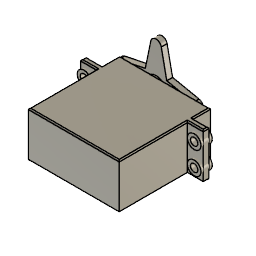
ASM of One of the legs (Autodesk Fusion 360 archive; units mm, degrees)
design "Servo MG996R Hosyond v2"
Autodesk Fusion 360 part; units mm, degrees
sketch "Sketch1" plane through (0, 0, 0) normal (0, 1, 0) x (1, 0, 0) in component "Servo Body"
  line L0 (20, 10) -> (-20, 10)
  line L1 (-20, 10) -> (-20, -10)
  line L2 (-20, -10) -> (20, -10)
  line L3 (20, -10) -> (20, 10)
  line L4 (20, 10) -> (-20, -10) construction
  line L5 (-20, 10) -> (20, -10) construction
  dimension "d20" = 40
  dimension "d21" = 20
  constraint horizontal L0
  constraint perpendicular L0 L1
  constraint parallel L0 L2
  constraint parallel L1 L3
  constraint coincident L4 origin
  constraint coincident L5 origin
  measures "d20" distance of L1.end L2.end
  measures "d21" distance of L0.end L1.end
extrude "Extrude1" add sketch "Sketch1" along normal blind 40.2 makes body 1 in component "Servo Body"
sketch "Sketch2" plane through (0, 40.2, 0) normal (0, 1, 0) x (-1, 0, 0) in component "Servo Body"
  line L0 (-20, 10) -> (-20, -10) construction
  line L1 (20, -10) -> (20, 10) construction
  line L2 (-20, 0) -> (20, 0) construction
  circle A0 centre (10, 0) radius 6.5
  circle A1 centre (10, 0) radius 2.9
  dimension "d24" = 10
  dimension "d25" = 13
  dimension "d26" = 5.8
  constraint midpoint L0 L2.start
  constraint midpoint L1 L2.end
  constraint coincident L2 A0.centre
  constraint concentric A0 A1
  measures "d24" distance of L2.end A0.centre
  measures "d25" diameter of A0
  measures "d26" diameter of A1
extrude "Extrude2" add sketch "Sketch2" along normal blind 2 contours A0 | A1 bodies 1 in component "Servo Body"
extrude "Extrude3" add sketch "Sketch2" along normal blind 6 contours A1 bodies 1 in component "Servo Body"
sketch "Sketch3" plane through (20, 0, 0) normal (1, 0, 0) x (0, 1, 0) in component "Servo Body"
  line L0 (30, 10) -> (32.5, 10)
  line L1 (32.5, 10) -> (32.5, -10)
  line L2 (32.5, -10) -> (30, -10)
  line L3 (30, -10) -> (30, 10)
  line L4 (0, 10) -> (40.2, 10)
  line L5 (0, -10) -> (40.2, -10)
  dimension "d31" = 2.5
  dimension "d32" = 30
  constraint horizontal L0
  constraint vertical L1
  constraint horizontal L2
  constraint vertical L3
  constraint coincident L1.end L5
  constraint coincident L0.start L4
  measures "d31" distance of L0.start L0.end
  measures "d32" distance of L0.start L4.start
extrude "Extrude4" add sketch "Sketch3" along normal blind 7 bodies 1 in component "Servo Body"
extrude "Extrude5" add sketch "Sketch3" against normal blind 7 from surface at -40 bodies 1 in component "Servo Body"
sketch "Sketch4" plane through (0, 32.5, 0) normal (0, 1, 0) x (-1, 0, 0) in component "Servo Body"
  circle A0 centre (24.25, -5) radius 2.22
  circle A1 centre (-24.25, -5) radius 2.22
  line L0 (20, -10) -> (27, -10)
  line L1 (20, 10) -> (27, 10)
  line L2 (-20, -10) -> (-27, -10)
  line L3 (-20, 10) -> (-27, 10)
  circle A2 centre (24.25, 5) radius 2.22
  circle A3 centre (-24.25, 5) radius 2.22
  line L4 (24.25, -5) -> (-24.25, -5) construction
  line L5 (-24.25, -5) -> (-24.25, 5) construction
  line L6 (-24.25, 5) -> (24.25, 5) construction
  line L7 (24.25, 5) -> (24.25, -5) construction
  line L8 (24.25, -5) -> (-24.25, 5) construction
  line L9 (-24.25, -5) -> (24.25, 5) construction
  line L10 (24.25, 0) -> (24.25, -10) construction
  dimension "d38" = 4.44
  dimension "d44" = 48.5
  constraint equal A0 A1
  constraint horizontal A0.centre A1.centre
  constraint equal A0 A2
  constraint equal A1 A3
  constraint horizontal L4
  constraint perpendicular L4 L5
  constraint parallel L4 L6
  constraint parallel L5 L7
  constraint coincident L8 origin
  constraint coincident L9 origin
  constraint coincident A0.centre L4.start
  constraint coincident A3.centre L5.end
  constraint coincident A2.centre L6.end
  constraint coincident A1.centre L4.end
  constraint midpoint L7 L10.start
  constraint coincident L0 L10.end
  constraint perpendicular L0 L10
  constraint midpoint A0.centre L10
  measures "d38" diameter of A0
  measures "d44" distance of A0.centre A1.centre
extrude "Extrude6" cut sketch "Sketch4" against normal up to surface (2.5 mm away) bodies 1 in component "Servo Body"
ref_plane "WorkPlane1" through (-10, 42.45, 0) normal (0, 1, 0) x (-1, 0, 0) in component "Connector"
sketch "Sketch1 (2)" plane through (0, 42.45, 0) normal (0, 1, 0) x (1, 0, 0) in component "Connector"
  arc A0 (-10, -18.3) -> (-7.6779, -16.4093) centre (-10, -15.9287) ccw
  line L0 (-5.2624, -4.7376) -> (-7.6779, -16.4093)
  line L1 (5.9287, 0) -> (6.4093, -2.3221) construction
  line L2 (-7.6779, -16.4093) -> (-10, -15.9287) construction
  arc A1 (6.4093, -2.3221) -> (8.3, 0) centre (5.9287, 0) ccw
  line L3 (-10, 0) -> (5.9287, 0) construction
  line L4 (6.4093, -2.3221) -> (-5.2624, -4.7376)
  line L5 (-5.2624, -4.7376) -> (-10, 0) construction
  line L6 (-10, -15.9287) -> (-10, -18.3) construction
  line L7 (5.9287, 0) -> (8.3, 0) construction
  line L8 (-10, -15.9287) -> (-10, 0) construction
  circle A2 centre (-10, 0) radius 4.35
  circle A3 centre (-10, 0) radius 2.9
  arc A4 (-28.3, 0) -> (-26.4093, -2.3221) centre (-25.9287, 0) ccw
  line L9 (-26.4093, -2.3221) -> (-14.7376, -4.7376)
  line L10 (-14.7376, -4.7376) -> (-12.3221, -16.4093)
  arc A5 (-12.3221, -16.4093) -> (-10, -18.3) centre (-10, -15.9287) ccw
  arc A6 (8.3, 0) -> (6.4093, 2.3221) centre (5.9287, 0) ccw
  line L11 (6.4093, 2.3221) -> (-5.2624, 4.7376)
  line L12 (-5.2624, 4.7376) -> (-7.6779, 16.4093)
  arc A7 (-7.6779, 16.4093) -> (-10, 18.3) centre (-10, 15.9287) ccw
  arc A8 (-10, 18.3) -> (-12.3221, 16.4093) centre (-10, 15.9287) ccw
  line L13 (-14.7376, 4.7376) -> (-12.3221, 16.4093)
  line L14 (-26.4093, 2.3221) -> (-14.7376, 4.7376)
  arc A9 (-26.4093, 2.3221) -> (-28.3, 0) centre (-25.9287, 0) ccw
  dimension "d2" = 6.7
  dimension "d3" = 45
  dimension "d5" = 18.3
  dimension "d7" = 2.3713
  dimension "d8" = 8.7
  constraint tangent A1 L4
  constraint coincident L1.start A1.centre
  constraint coincident A0.centre L2.end
  constraint equal L6 L7
  constraint tangent A0 L0
  constraint vertical L8
  constraint horizontal L3
  constraint vertical L6
  constraint horizontal L7
  constraint equal L3 L8
  constraint coincident L3.start L5.end
  constraint symmetric A1.end L8 A4.start
  constraint symmetric A0.end L8 L10.end
  constraint symmetric A0.start L8 L6.end
  constraint symmetric L1.end L8 A4.end
  constraint symmetric L0.start L8 L9.end
  constraint symmetric A0 L8 A5
  constraint symmetric A1 L8 A4
  constraint symmetric A1.end L3 L7.end
  constraint symmetric A0.end L3 L12.end
  constraint symmetric A0.start L3 A7.end
  constraint symmetric L1.end L3 A6.end
  constraint symmetric L0.start L3 L11.end
  constraint symmetric A0 L3 A7
  constraint symmetric A1 L3 A6
  constraint symmetric L3 A4.end L14.start
  constraint symmetric L3 A4.start A9.end
  constraint symmetric L3 A4 A9
  constraint symmetric L3 L9.end L13.start
  constraint symmetric L3 L10.end A8.end
  constraint symmetric L3 A0.start A7.end
  constraint symmetric L3 A5 A8
  measures "d2" distance of L3.start L0.start
  measures "d3" angle of L3 L5
  measures "d5" distance of L3.start A0.start
  measures "d7" distance of A0.end A0.centre
  measures "d8" diameter of A2
extrude "Extrude1'" add sketch "Sketch1 (2)" along normal blind 3 separate body contours A2 makes body 2 in component "Connector"
extrude "Extrude2'" add sketch "Sketch1 (2)" along normal blind 2.6 from surface at 3 separate body contours A0 L0 A1 L4 A4 L9 L10 A5 A6 L11 L12 A7 A8 L13 L14 A9 | A2 makes body 3 in component "Connector"
ref_plane "WorkPlane1" through (23.5, 31.25, 0) normal (0, -1, 0) x (0, 0, -1) in component "Rubber Feet"
sketch "Sketch1 (3)" plane through (0, 31.25, 0) normal (0, -1, 0) x (-1, 0, 0) in component "Rubber Feet"
  circle A0 centre (-24.25, -5) radius 3
  circle A1 centre (-24.25, -5) radius 1.625
  circle A2 centre (-24.25, 5) radius 1.625
  circle A3 centre (-24.25, 5) radius 3
  circle A4 centre (24.25, -5) radius 1.625
  circle A5 centre (24.25, -5) radius 3
  circle A6 centre (24.25, 5) radius 1.625
  circle A7 centre (24.25, 5) radius 3
  circle A8 centre (-24.25, 5) radius 2.22
  circle A9 centre (-24.25, -5) radius 2.22
  circle A10 centre (24.25, 5) radius 2.22
  circle A11 centre (24.25, -5) radius 2.22
  dimension "d14" = 6
  dimension "d15" = 3.25
  constraint equal A1 A2
  constraint equal A4 A6
  constraint equal A0 A3
  constraint equal A5 A7
  constraint equal A0 A5
  constraint equal A1 A4
  constraint coincident A6.centre A7.centre
  constraint coincident A4.centre A5.centre
  constraint coincident A2.centre A3.centre
  constraint coincident A0.centre A1.centre
  measures "d14" diameter of A0
  measures "d15" diameter of A1
extrude "Extrude1''" add sketch "Sketch1 (3)" along normal blind 2.5 and the other way blind 2.5 separate body contours A0 | A3 | A5 | A7 | A8 | A9 | A10 | A11 makes body 4 at (21.2537, 29.5833, -4.8505) makes body 5 at (-27.2463, 29.5833, 5.1495) makes body 6 at (21.2537, 29.5833, 5.1495) makes body 7 at (-27.2463, 29.5833, -4.8505) in component "Rubber Feet"
fillet "Fillet1" radius 0.5 2 faces at (6.6667, 10, 10) (6.6667, 20, -10) on bodies 1 in component "Servo Body"
other "GeometricRelationship1"
other "GeometricRelationship4"
other "GeometricRelationship5"
component "Connector" placed x (1, 0, 0) y (0, 1, 0) z (0, 0, 1) at (0, 0.75, 0)
component "Servo Body" placed x (1, 0, 0) y (0, 1, 0) z (0, 0, 1) at (0, 0, 0)
component "Rubber Feet" placed x (1, 0, 0) y (0, 1, 0) z (0, 0, 1) at (0, 0, 0)

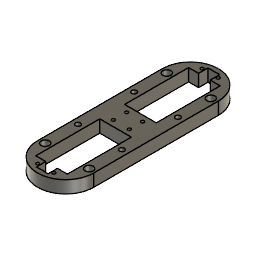
design "Shin"
Autodesk Fusion 360 part; units mm, degrees
sketch "Sketch1" plane through (0, 0, 0) normal (0, 0, 1) x (1, 0, 0)
  line L0 (18, 0) -> (18, 40)
  line L1 (18, 40) -> (-18, 40)
  line L2 (-18, 40) -> (-18, 0)
  arc A0 (18, 40) -> (-18, 40) centre (0, 40) ccw
  line L3 (-10.15, 8) -> (10.15, 8)
  line L4 (10.15, 8) -> (10.15, 49)
  line L5 (-10.15, 49) -> (-10.15, 8)
  line L6 (3.75, 49) -> (3.75, 55)
  line L7 (3.75, 55) -> (-3.75, 55)
  line L8 (-3.75, 55) -> (-3.75, 49)
  line L9 (10.15, 49) -> (3.75, 49)
  line L10 (-3.75, 49) -> (-10.15, 49)
  circle A1 centre (5.15, 52.75) radius 1
  line L11 (0, 55) -> (0, 40)
  line L12 (10.15, 28.5) -> (-10.15, 28.5)
  circle A2 centre (-5.15, 52.75) radius 1
  circle A3 centre (-5.15, 4.25) radius 1
  circle A4 centre (5.15, 4.25) radius 1
  line L13 (-18, 0) -> (18, 0)
  circle A5 centre (-5.15, -52.75) radius 1
  circle A6 centre (5.15, -4.25) radius 1
  line L14 (-10.15, -8) -> (10.15, -8)
  line L15 (18, 0) -> (18, -40)
  circle A7 centre (5.15, -52.75) radius 1
  line L16 (-10.15, -49) -> (-10.15, -8)
  circle A8 centre (-5.15, -4.25) radius 1
  line L17 (0, -55) -> (0, -40)
  line L18 (3.75, -49) -> (3.75, -55)
  line L19 (18, -40) -> (-18, -40)
  line L20 (-3.75, -55) -> (-3.75, -49)
  line L21 (10.15, -28.5) -> (-10.15, -28.5)
  line L22 (10.15, -8) -> (10.15, -49)
  line L23 (3.75, -55) -> (-3.75, -55)
  line L24 (10.15, -49) -> (3.75, -49)
  line L25 (-18, -40) -> (-18, 0)
  line L26 (-3.75, -49) -> (-10.15, -49)
  arc A9 (-18, -40) -> (18, -40) centre (0, -40) ccw
  point P0 (0, 40)
  point P1 (0, 8)
  point P2 (0, 55)
  point P3 (0, -55)
  point P4 (0, -8)
  point P5 (0, -40)
  dimension "d1" = 40
  dimension "d2" = 36
  dimension "d3" = 41
  dimension "d4" = 20.3
  dimension "d5" = 7.5
  dimension "d6" = 6
  dimension "d7" = 2
  dimension "d8" = 5
  dimension "d9" = 3.75
  dimension "d10" = 15
  constraint vertical L0
  constraint horizontal L1
  constraint vertical L2
  constraint midpoint L1 P0
  constraint vertical origin A0.centre
  constraint coincident P0 A0.centre
  constraint horizontal L3
  constraint vertical L4
  constraint horizontal L9
  constraint vertical L5
  constraint midpoint L3 P1
  constraint vertical origin P1
  constraint vertical L6
  constraint horizontal L7
  constraint vertical L8
  constraint coincident L8.end L9
  constraint collinear L9 L10
  constraint midpoint L7 P2
  constraint vertical P1 P2
  constraint coincident P2 L11.start
  constraint midpoint L4 L12.start
  constraint midpoint L5 L12.end
  constraint symmetric A1 L11 A2
  constraint symmetric A1 L12 A4
  constraint symmetric L12 A2 A3
  constraint horizontal L2.end origin
  constraint perpendicular L0 L13
  constraint symmetric L2.end L13 L25.end
  constraint symmetric L0.start L13 L15.start
  constraint symmetric L0.end L13 L15.end
  constraint symmetric L1.end L13 L19.end
  constraint symmetric P0 L13 L17.end
  constraint symmetric A0 L13 A9
  constraint symmetric L3.start L13 L14.start
  constraint symmetric L3.end L13 L14.end
  constraint symmetric L4.end L13 L22.end
  constraint symmetric L5.start L13 L16.start
  constraint symmetric P1 L13 P4
  constraint symmetric L8.end L13 L20.end
  constraint symmetric L6.start L13 L18.start
  constraint symmetric L6.end L13 L18.end
  constraint symmetric L7.end L13 L20.start
  constraint symmetric P2 L13 P3
  constraint symmetric A1 L13 A7
  constraint symmetric P0 L13 P5
  constraint symmetric L12.start L13 L21.start
  constraint symmetric L12.end L13 L21.end
  constraint symmetric A2 L13 A5
  constraint symmetric A3 L13 A8
  constraint symmetric A4 L13 A6
  measures "d1" distance of L2.end L1.end
  measures "d2" distance of L0 L2
  measures "d3" distance of L3.start L5.start
  measures "d4" distance of L3.start L3.end
  measures "d5" distance of L6.end L7.end
  measures "d6" distance of L8.end L7.end
  measures "d7" diameter of A1
  measures "d8" horizontal distance of L4.end A1.centre
  measures "d9" vertical distance of L4.end A1.centre
  measures "d10" distance of P2 P0
extrude "Extrude1" add sketch "Sketch1" along normal blind 8 contours L0 L1 L2 L3 L4 L5 L13 | L13 L14 L15 L16 L19 L22 L25 | L1 A0 L4 L5 L6 L7 L8 L9 L10 | L16 L18 L19 L20 L22 L23 L24 L26 A9
sketch "Sketch2" plane through (0, 0, 8) normal (0, 0, 1) x (-1, 0, 0)
  circle A0 centre (-5.15, -4.25) radius 1
  circle A1 centre (-5.15, -52.75) radius 1
  circle A2 centre (5.15, -52.75) radius 1
  line L0 (10.15, -49) -> (3.75, -49)
  line L1 (3.75, -49) -> (3.75, -55)
  line L2 (3.75, -55) -> (-3.75, -55)
  line L3 (-3.75, -55) -> (-3.75, -49)
  line L4 (-3.75, -49) -> (-10.15, -49)
  line L5 (-10.15, -49) -> (-10.15, -8)
  line L6 (-10.15, -8) -> (10.15, -8)
  line L7 (10.15, -8) -> (10.15, -49)
  circle A3 centre (5.15, -4.25) radius 1
  line L8 (-18, 40) -> (-18, -40)
  arc A4 (-18, -40) -> (18, -40) centre (0, -40) ccw
  line L9 (18, -40) -> (18, 40)
  circle A5 centre (14.075, -39) radius 1.6
  circle A6 centre (14.075, -39) radius 2.6
  line L10 (18, -39) -> (10.15, -39)
  line L11 (0, -55) -> (0, -8)
  line L12 (10.15, -28.5) -> (-10.15, -28.5)
  circle A7 centre (14.075, -18) radius 2.6
  circle A8 centre (14.075, -18) radius 1.6
  circle A9 centre (-14.075, -39) radius 1.6
  circle A10 centre (-14.075, -39) radius 2.6
  circle A11 centre (-14.075, -18) radius 1.6
  circle A12 centre (-14.075, -18) radius 2.6
  circle A13 centre (-5.15, 52.75) radius 1
  line L13 (3.75, 55) -> (3.75, 49)
  line L14 (3.75, 49) -> (10.15, 49)
  line L15 (10.15, 49) -> (10.15, 8)
  line L16 (10.15, 8) -> (-10.15, 8)
  line L17 (-10.15, 8) -> (-10.15, 49)
  line L18 (-10.15, 49) -> (-3.75, 49)
  line L19 (-3.75, 49) -> (-3.75, 55)
  line L20 (-3.75, 55) -> (3.75, 55)
  circle A14 centre (5.15, 52.75) radius 1
  circle A15 centre (5.15, 4.25) radius 1
  circle A16 centre (-5.15, 4.25) radius 1
  arc A17 (18, 40) -> (-18, 40) centre (0, 40) ccw
  line L21 (18, 0) -> (-18, 0)
  circle A18 centre (14.075, 18) radius 2.6
  circle A19 centre (14.075, 18) radius 1.6
  circle A20 centre (14.075, 39) radius 1.6
  circle A21 centre (14.075, 39) radius 2.6
  circle A22 centre (-14.075, 39) radius 1.6
  circle A23 centre (-14.075, 39) radius 2.6
  circle A24 centre (-14.075, 18) radius 1.6
  circle A25 centre (-14.075, 18) radius 2.6
  point P0 (14.075, -39)
  dimension "d25" = 3.2
  dimension "d26" = 5.2
  dimension "d28" = 10
  constraint concentric A5 A6
  constraint coincident L9 L10.start
  constraint coincident L7 L10.end
  constraint perpendicular L7 L10
  constraint midpoint L10 P0
  constraint coincident P0 A5.centre
  constraint midpoint L2 L11.start
  constraint midpoint L6 L11.end
  constraint midpoint L7 L12.start
  constraint midpoint L5 L12.end
  constraint symmetric A5 L12 A8
  constraint symmetric A6 L12 A7
  constraint symmetric A5 L11 A9
  constraint symmetric A6 L11 A10
  constraint symmetric L11 A7 A12
  constraint symmetric L11 A8 A11
  constraint midpoint L9 L21.start
  constraint midpoint L8 L21.end
  constraint symmetric A5 L21 A20
  constraint symmetric A6 L21 A21
  constraint symmetric A7 L21 A18
  constraint symmetric A8 L21 A19
  constraint symmetric A9 L21 A22
  constraint symmetric A10 L21 A23
  constraint symmetric A11 L21 A24
  constraint symmetric A12 L21 A25
  measures "d25" diameter of A5
  measures "d26" diameter of A6
  measures "d28" distance of L0.start L10.end
extrude "Extrude2" cut sketch "Sketch2" against normal up to surface (8 mm away) contours A5 L10 | A5 L10 | A8 | A9 | A11 | A19 | A20 | A22 | A24
extrude "Extrude3" cut sketch "Sketch2" against normal blind 4 contours A5 A6 L10 | A5 A6 L10 | A10 | A21 | A23
sketch "Sketch3" plane through (0, 0, 0) normal (0, 0, 1) x (-1, 0, 0)
  circle A0 centre (-14.075, -18) radius 1.6
  circle A1 centre (14.075, 18) radius 1.6
  circle A2 centre (14.075, -18) radius 1.6
  circle A3 centre (-14.075, 18) radius 1.6
  circle A4 centre (-14.075, -39) radius 1.6
  circle A5 centre (14.075, 39) radius 1.6
  circle A6 centre (14.075, -39) radius 1.6
  circle A7 centre (-14.075, 39) radius 1.6
  circle A8 centre (-5.15, -4.25) radius 1
  circle A9 centre (-5.15, -52.75) radius 1
  circle A10 centre (-5.15, 52.75) radius 1
  circle A11 centre (5.15, -4.25) radius 1
  line L0 (3.75, 49) -> (3.75, 55)
  line L1 (3.75, 55) -> (-3.75, 55)
  line L2 (-3.75, 55) -> (-3.75, 49)
  line L3 (-3.75, 49) -> (-10.15, 49)
  line L4 (-10.15, 49) -> (-10.15, 8)
  line L5 (-10.15, 8) -> (10.15, 8)
  line L6 (10.15, 8) -> (10.15, 49)
  line L7 (10.15, 49) -> (3.75, 49)
  circle A12 centre (5.15, -52.75) radius 1
  circle A13 centre (5.15, 52.75) radius 1
  circle A14 centre (5.15, 4.25) radius 1
  circle A15 centre (-5.15, 4.25) radius 1
  line L8 (3.75, -49) -> (10.15, -49)
  line L9 (10.15, -49) -> (10.15, -8)
  line L10 (10.15, -8) -> (-10.15, -8)
  line L11 (-10.15, -8) -> (-10.15, -49)
  line L12 (-10.15, -49) -> (-3.75, -49)
  line L13 (-3.75, -49) -> (-3.75, -55)
  line L14 (-3.75, -55) -> (3.75, -55)
  line L15 (3.75, -55) -> (3.75, -49)
  line L16 (-18, -40) -> (-18, 40)
  arc A16 (18, 40) -> (-18, 40) centre (0, 40) ccw
  line L17 (18, 40) -> (18, -40)
  arc A17 (-18, -40) -> (18, -40) centre (0, -40) ccw
  circle A18 centre (-14.075, -18) radius 2.6
  circle A19 centre (-14.075, 18) radius 2.6
  circle A20 centre (14.075, 18) radius 2.6
  circle A21 centre (14.075, -18) radius 2.6
extrude "Extrude4" cut sketch "Sketch3" along normal blind 4 contours A18 | A19 | A20 | A21
